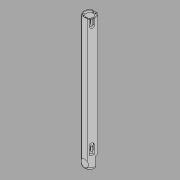
# Autodesk Inventor part: inner leg
Saved by Autodesk Inventor 2020 (Build 240168000, 168)
## iProperties
Created: 2020-12-28
Part Number: inner leg
Material: Generic
Document SubType Name: Modeling
Designer: freyja
Density: 1 g/cm^3
Appearance: Default
Author: freyja
Autodesk Inventor part; units mm, degrees
ref_plane "YZ Plane" through (0, 0, 0) normal (1, 0, 0) x (0, 1, 0)
sketch "Sketch1" plane through (0, 0, 0) normal (0, 1, 0) x (-1, 0, 0)
  circle A0 centre (0, 0) radius 3.5
  dimension "d0" = 7
  constraints: 1 centre point, 1 coincident
  measures "d0" diameter of A0
extrude "Extrusion1" add sketch "Sketch1" along normal blind 70
ref_plane "Work Plane1" through (0, 35, 0) normal (0, -1, 0) x (1, 0, 0)
ref_plane "Work Plane2" through (0, 0, -3.5) normal (0, 0, 1) x (1, 0, 0)
sketch "Sketch4" plane through (0, 0, -3.5) normal (0, 0, 1) x (1, 0, 0)
  line L0 (0, 66) -> (0, 70) construction
  line L1 (1.25, 66) -> (1.25, 70)
  line L2 (-1.25, 70) -> (-1.25, 66)
  arc A0 (-1.25, 66) -> (1.25, 66) centre (0, 66) ccw
  arc A1 (1.25, 70) -> (-1.25, 70) centre (0, 70) ccw
  line L3 (3.5, 70) -> (-3.5, 70) projected
  line L4 (0, 70) -> (0, 69.1822)
  point P0 (0, 0)
  point P1 (0, 68)
  point P2 (1.25, 70)
  point P3 (-1.25, 70)
  point P4 (1.25, 70)
  point P5 (-1.25, 70)
  dimension "d17" = 2.5
  dimension "d18" = 4
  constraints: 10 end point, 4 point on circle, 4 tangent, 3 midpoint, 2 centre point, 2 vertical, 1 collinear, 1 parallel
  measures "d17" diameter of A1
  measures "d18" distance of L0.start L0.end
extrude "Extrusion3" cut sketch "Sketch4" along normal blind 1 draft -20
sketch "Sketch5" plane through (0, 0, -2.5) normal (0, 0, -1) x (-1, 0, 0)
  line L0 (0, 69) -> (0, 67) construction
  line L1 (-0.5, 69) -> (-0.5, 67)
  line L2 (0.5, 67) -> (0.5, 69)
  arc A0 (0.5, 69) -> (-0.5, 69) centre (0, 69) ccw
  arc A1 (-0.5, 67) -> (0.5, 67) centre (0, 67) ccw
  line L3 (-0.886, 70) -> (0.886, 70) projected
  line L4 (3.5, 70) -> (-3.5, 70) projected
  line L5 (0, 70) -> (0, 68.8597)
  point P0 (0, 0)
  point P1 (0, 68)
  point P2 (1.1759, 70)
  point P3 (-1.1759, 70)
  dimension "d21" = 1
  dimension "d22" = 2
  dimension "d23" = 1
  constraints: 10 end point, 4 point on circle, 4 tangent, 2 centre point, 2 midpoint, 2 vertical, 1 parallel, 1 point on line
  measures "d21" diameter of A1
  measures "d22" distance of L0.start L0.end
  measures "d23" distance from line of L3 L0.start
extrude "Extrusion4" add sketch "Sketch5" along normal blind 1
pattern_circular "Circular Pattern1" count 3 over 360 about axis through (0, -10, 0) along (0, 1, 0) of "Extrusion3", "Extrusion4"
sketch "Sketch6" plane through (0, 0, 0) normal (1, 0, 0) x (0, 1, 0)
  line L0 (69.5, -2.5) -> (69, -2.5) projected
  circle A0 centre (69.5, -2.5) radius 0.5
  line L1 (-15.2, 0) -> (84.2, 0) projected
  point P0 (0, 0)
  constraints: 1 centre point
revolve "Revolution1" cut sketch "Sketch6" angle 360 about axis through (0, -10, 0) along (0, 1, 0)
sketch "Sketch7" plane through (0, 70, 0) normal (0, 1, 0) x (1, 0, 0)
  circle A0 centre (0, 0) radius 5
  dimension "d30" = 10
  constraints: 1 centre point, 1 coincident
  measures "d30" diameter of A0
extrude "Extrusion5" cut sketch "Sketch7" against normal blind 0.3
sketch "Sketch8" plane through (0, 69.7, 0) normal (0, 1, 0) x (1, 0, 0)
  circle A0 centre (0, 0) radius 2.5
  dimension "d33" = 5
  constraints: 1 centre point, 1 coincident
  measures "d33" diameter of A0
extrude "Extrusion6" cut sketch "Sketch8" against normal blind 0.5
mirror "Mirror2" about plane through (0, 35, 0) normal (0, -1, 0) of "Extrusion3", "Extrusion4", "Circular Pattern1", "Revolution1", "Extrusion5", "Extrusion6"
sketch "Sketch9" plane through (0, 0.8, 0) normal (0, -1, 0) x (1, 0, 0)
  circle A0 centre (0, 0) radius 2.1 projected
  arc A1 (1.1759, -3.2965) -> (3.4429, 0.6299) centre (0, 0) ccw projected
  arc A2 (2.2669, 2.6667) -> (-2.2669, 2.6667) centre (0, 0) ccw projected
  arc A3 (-3.4429, 0.6299) -> (-1.1759, -3.2965) centre (0, 0) ccw projected
  arc A4 (2.2669, 2.6667) -> (-2.2669, 2.6667) centre (0, 0) ccw projected
  arc A5 (1.1759, -3.2965) -> (3.4429, 0.6299) centre (0, 0) ccw projected
  arc A6 (-3.4429, 0.6299) -> (-1.1759, -3.2965) centre (0, 0) ccw projected
  arc A7 (-3.4429, 0.6299) -> (-1.1759, -3.2965) centre (0, 0) ccw projected
  line L0 (-1.1759, -3.2965) -> (-0.6971, -1.9809)
  line L1 (-1.1759, -3.2965) -> (-0.886, -2.5) projected
  line L2 (1.1759, -3.2965) -> (0.886, -2.5) projected
  line L3 (1.1759, -3.2965) -> (0.6971, -1.9809)
  line L4 (-3.4429, 0.6299) -> (-2.6081, 0.4827) projected
  line L5 (-3.4429, 0.6299) -> (-2.0641, 0.3868)
  circle A8 centre (0, 0) radius 2.1 projected
  line L6 (-2.2669, 2.6667) -> (-1.722, 2.0173) projected
  line L7 (-1.367, 1.5942) -> (-2.2669, 2.6667)
  line L8 (2.2669, 2.6667) -> (1.367, 1.5942)
  line L9 (2.2669, 2.6667) -> (1.722, 2.0173) projected
  line L10 (3.4429, 0.6299) -> (2.6081, 0.4827) projected
  line L11 (3.4429, 0.6299) -> (2.0641, 0.3868)
  point P0 (2.2669, 2.6667)
  constraints: 12 end point, 6 collinear, 6 point on circle, 12 other
extrude "Extrusion7" add sketch "Sketch9" along normal blind 2
sketch "Sketch12" plane through (0, -1.2, 0) normal (0, -1, 0) x (1, 0, 0)
  circle A0 centre (0, 0) radius 3.5
  constraints: 1 centre point, 1 coincident
extrude "Extrusion9" add sketch "Sketch12" along normal blind 8
sketch "Sketch13" plane through (0, -9.2, 0) normal (0, -1, 0) x (1, 0, 0)
  circle A0 centre (0, 0) radius 3.5 projected
  line L0 (3.5, 0) -> (-3.5, 0)
  arc A1 (2.2669, 2.6667) -> (-2.2669, 2.6667) centre (0, 0) ccw projected
  line L1 (1.6248, 3.1) -> (-1.6248, 3.1)
  point P0 (-1.6248, 3.1)
  dimension "d53" = 3.1
  constraints: 4 end point, 4 point on circle, 1 horizontal, 1 midpoint, 1 parallel
  measures "d53" distance between parallel lines of L0 L1
extrude "Extrusion10" cut sketch "Sketch13" against normal blind 7 contours A0 L0 | L1 A0
sketch "Sketch14" plane through (3.5, -9.2, 0) normal (0, 0, -1) x (-1, 0, 0)
  line L0 (7, 0) -> (0, 0) projected
  line L1 (7, 7) -> (7, 0) projected
  point P0 (3.5, 9.2)
  point P1 (3.5, 3)
  dimension "d56" = 3
  dimension "d57" = 7
  dimension "d58" = 3.5
  measures "d56" distance from line of L0 point (3.5, 3)
  measures "d57" distance of L0.start L0.end
  measures "d58" distance from line of L1 point (3.5, 3)
hole "Hole2" at (0, -6.2, 0) direction (0, 0, 1) diameter 4.305 end through all clearance for "Flat Head Machine Screw (82)" size "#8" standard "Ansi Unified Screw Threads"
fillet "Fillet3" radius 1.5 1 edges at (2.9947, -9.2, 1.8115)
sketch "Sketch15" plane through (0, -2.2, 0) normal (0, -1, 0) x (1, 0, 0)
  line L0 (1.6248, 3.1) -> (-1.6248, 3.1) projected
  arc A0 (1.6248, 3.1) -> (-1.6248, 3.1) centre (0, 0) ccw projected
extrude "Extrusion11" cut sketch "Sketch15" against normal through all
ref_plane "Work Plane3" through (0, 70, -3.5) normal (0, 0, -1) x (1, 0, 0)
equation "\"d58\" = 0.5 * d57"
body "Solid1"
